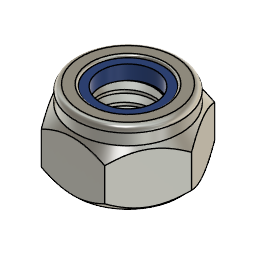
M6_nylock_hex_nut (Autodesk Fusion 360 design; units mm, degrees)
part number: 2026-04-25-09-47-30-495
Autodesk Fusion 360 part; units mm, degrees
sketch "Hex Nut Shape" plane through (0, 0, 0) normal (0, 0, 1) x (1, 0, 0)
  line L0 (-2.8868, 5) -> (-5.7735, 0)
  line L1 (-5.7735, 0) -> (-2.8868, -5)
  line L2 (-2.8868, -5) -> (2.8868, -5)
  line L3 (2.8868, -5) -> (5.7735, 0)
  line L4 (5.7735, 0) -> (2.8868, 5)
  line L5 (2.8868, 5) -> (-2.8868, 5)
  dimension "d3" = 10
  measures "d3" distance of L2 L5
extrude "Extrude1" add sketch "Hex Nut Shape" along normal blind 5 makes body 1
sketch "Chamfer Outline" plane through (0, 0, 0) normal (0, 1, 0) x (1, 0, 0)
  line L0 (2.8868, 0) -> (5.7735, 0)
  line L1 (5.7735, 0) -> (5.7735, -5)
  line L2 (5.7735, -5) -> (2.8868, -5)
  line L3 (2.8868, -5) -> (2.8868, 0)
  line L4 (-2.8868, 0) -> (2.8868, 0)
  line L5 (2.8868, 0) -> (2.8868, -5)
  line L6 (2.8868, -5) -> (-2.8868, -5)
  line L7 (-2.8868, -5) -> (-2.8868, 0)
  line L8 (-5.7735, 0) -> (-2.8868, 0)
  line L9 (-2.8868, 0) -> (-2.8868, -5)
  line L10 (-2.8868, -5) -> (-5.7735, -5)
  line L11 (-5.7735, -5) -> (-5.7735, 0)
  line L12 (5.7735, -5) -> (4.7735, -5)
  line L13 (5.7735, -5) -> (5.7735, -4)
  line L14 (5.7735, 0) -> (5.7735, -1)
  line L15 (5.7735, 0) -> (4.7735, 0)
  line L16 (4.7735, -5) -> (5.7735, -4)
  line L17 (5.7735, -1) -> (4.7735, 0)
  dimension "d11" = 1
  dimension "d12" = 1
  dimension "d13" = 1
  dimension "d14" = 1
  constraint coincident L1.end L2.start
  constraint perpendicular L1 L12
  constraint coincident L1 L13.end
  constraint coincident L0.end L1.start
  constraint perpendicular L2 L14
  constraint perpendicular L14 L15
  measures "d11" distance of L1.end L12.end
  measures "d12" distance of L1.end L13.end
  measures "d13" distance of L0.end L14.end
  measures "d14" distance of L0.end L15.end
revolve "Revolve1" cut sketch "Chamfer Outline" angle 360 about axis through (0, 0, 1.75) along (0, 0, 1) contours L0 L1 L14 L15 L17 | L1 L2 L12 L13 L16 bodies 1
hole "Hole1" at (0, 0, 5) direction (0, 0, -1) diameter 6 end through all bodies 1
chamfer "Chamfer1" distance 0.25 angle 45 1 edges at (-2.797, -1.0848, 0) on bodies 1
thread "Thread1" "ISO Metric profile 6.0 M6x1 M6x1 6H" major diameter 6.147 minor diameter 5.035 pitch 1 angle 60 modelled right hand crest width 0.2748 on face at (0.2987, -2.9851, 3.4167) crest through (2.5175, 0, 4.75) on bodies 1
sketch "Nylock Outline" plane through (0, 0, 5) normal (0, 0, 1) x (-1, 0, 0)
  spline S0 degree 3 poles (0.7938, 2.9692) (1.1619, 2.8346) (1.5007, 2.6305) (2.069, 2.1114) (2.2965, 1.8052) (2.6132, 1.1343) (2.704, 0.7783) (2.7408, 0.0652) (2.6916, -0.2847) (2.5067, -0.8107) (2.4149, -0.9977) (2.1912, -1.3413) (2.061, -1.4974) (1.9135, -1.636) knots 0 0 0 0 0.117588 0.117588 0.231087 0.231087 0.340498 0.340498 0.445817 0.445817 0.508297 0.508297 0.569249 0.569249 0.569249 0.569249
  arc A0 (-1.9135, -1.636) -> (1.9135, -1.636) centre (0, 0) ccw
  spline S1 degree 3 poles (-1.9135, -1.636) (-2.1558, -1.4082) (-2.3504, -1.1345) (-2.6319, -0.5162) (-2.7113, -0.1755) (-2.7381, 0.5311) (-2.68, 0.8904) (-2.4271, 1.5805) (-2.2298, 1.9028) (-1.817, 2.3542) (-1.6364, 2.5092) (-1.2382, 2.776) (-1.0214, 2.886) (-0.7938, 2.9692) knots 0 0 0 0 0.09977 0.09977 0.203618 0.203618 0.311544 0.311544 0.423544 0.423544 0.494428 0.494428 0.566847 0.566847 0.566847 0.566847
  arc A1 (0.7938, 2.9692) -> (-0.7938, 2.9692) centre (0, 0) ccw
  circle A2 centre (0, 0) radius 4.7735
  circle A3 centre (0, 0) radius 2.5
  circle A4 centre (0, 0) radius 3.2
  dimension "d23" = 5
  dimension "d24" = 0.7
  constraint concentric A0 A3
  constraint concentric A0 A4
  measures "d23" diameter of A3
  measures "d24" distance of A3 A4
extrude "Extrude2" add sketch "Nylock Outline" along normal blind 1.3 separate body contours S0 A0 S1 A1 | A4 makes body 2
extrude "Extrude3" add sketch "Nylock Outline" along normal blind 1.5 contours A2 bodies 1
fillet "Fillet2" radius 0.5 1 edges at (4.4505, 1.7262, 6.5) on bodies 1
fillet "Fillet3" radius 0.2 1 edges at (2.9834, -1.1572, 6.5) on bodies 1
equation "width_across_flats = 10 mm" comment "An M6 hex nut has a widths across the flats of 10 mm."
equation "thickness = 5 mm" comment "An M6 hex nut has a thickness of 5 mm."
equation "d3 = width_across_flats"
equation "d4 = thickness"
equation "chamfer_side_length = 1 mm" comment "Chamfer on the outside top and bottom of the hex nut."
equation "d11 = chamfer_side_length"
equation "d12 = chamfer_side_length"
equation "d13 = chamfer_side_length"
equation "d14 = chamfer_side_length"
equation "d16 = hole_diameter"
equation "hole_diameter = 6 mm" comment "An M6 hex nut has a hole diameter of 6 mm."
equation "hole_chamfer = 0.25 mm" comment "Chamfer on the inside of the hex nut thread hole."
equation "d20 = hole_chamfer"
equation "d23 = hole_diameter - 1 mm"
equation "d24 = nylon_thickness"
equation "nylon_thickness = 0.7 mm" comment "The thickness of the nylon insert for the Nylock hex nut."
equation "top_height = 1.5 mm" comment "The height of the top portion containing the nylon insert."
equation "d27 = nylon_height"
equation "d29 = top_height"
equation "d35 = top_outside_fillet_radius"
equation "top_outside_fillet_radius = 0.5 mm" comment "The radius of the fillet on the outside of the top portion containing the nylon insert."
equation "nylon_height = top_height - top_inside_fillet_radius" comment "The height of the nylon insert for the Nylock hex nut."
equation "top_inside_fillet_radius = 0.2 mm" comment "The radius of the fillet on the inside of the top portion containing the nylon insert."
equation "d40 = top_inside_fillet_radius"
named bodies: "M6 Hex Nut", "Nylon Insert"
